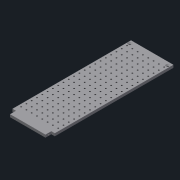
# Autodesk Inventor part: Mounting plate
Saved by Autodesk Inventor 2021.1 (Build 251245000, 245)
## iProperties
Created: 2020-05-07
Part Number: Mounting plate
Material: Generic
Document SubType Name: Modeling
Designer: Workshop Tech
Density: 1 g/cm^3
Appearance: Default
Author: Workshop Tech
Autodesk Inventor part; units mm, degrees
ref_plane "YZ Plane" through (0, 0, 0) normal (1, 0, 0) x (0, 1, 0)
ref_plane "XZ Plane" through (0, 0, 0) normal (0, 1, 0) x (-1, 0, 0)
ref_plane "XY Plane" through (0, 0, 0) normal (0, 0, 1) x (1, 0, 0)
sketch "Sketch1" plane through (0, 0, 0) normal (0, 1, 0) x (-1, 0, 0)
  line L0 (0, 0) -> (101.6, 0)
  line L1 (101.6, 0) -> (101.6, -298.45)
  line L2 (101.6, -298.45) -> (0, -298.45)
  line L3 (0, -298.45) -> (0, 0)
  dimension "d0" = 101.6
  dimension "d1" = 298.45
  constraints: 8 end point, 2 parallel, 1 horizontal, 1 perpendicular
  measures "d0" distance between parallel lines of L3 L1
  measures "d1" distance between parallel lines of L2 L0
extrude "Base" add sketch "Sketch1" along normal blind 6.35
sketch "Sketch7" plane through (0, 6.35, 0) normal (0, 1, 0) x (1, 0, 0)
  line L0 (0, 0) -> (0, 298.45) projected
  line L1 (-101.6, 0) -> (0, 0) projected
  line L2 (-101.6, 0) -> (0, 0) projected
  line L3 (0, 0) -> (0, 298.45) projected
  line L4 (0, 298.45) -> (-101.6, 298.45) projected
  line L5 (-101.6, 298.45) -> (-101.6, 0) projected
  point P0 (-95.25, 282.575)
  dimension "d35" = 15.875
  dimension "d36" = 6.35
  measures "d35" distance from line of L4 point (-95.25, 282.575)
  measures "d36" distance from line of L5 point (-95.25, 282.575)
hole "Threaded Mount Holes" at (-95.25, 6.35, -282.575) direction (0, -1, 0) diameter 3.242 end through all thread size "M4x0.7" class "6H" standard "ANSI Metric M Profile"
pattern_linear "Threaded Holes" count 21 spacing 12.7 along (0, 0, 1) count 8 spacing 12.7 along (1, 0, 0) of "Threaded Mount Holes"
sketch "Sketch8" plane through (0, 6.35, 0) normal (0, 1, 0) x (1, 0, 0)
  line L0 (0, 298.45) -> (-101.6, 298.45) projected
  line L1 (-101.6, 298.45) -> (-101.6, 0) projected
  point P0 (0, 0)
  point P1 (-96.4184, 290.703)
  dimension "d50" = 7.747
  dimension "d51" = 5.1816
  measures "d50" distance from line of L0 point (-96.418, 290.703)
  measures "d51" distance from line of point (-96.418, 290.703) L1
hole "Leg Mount Holes" at (-96.4184, 6.35, -290.703) direction (0, -1, 0) diameter 4.2926 end through all countersink diameter 9.398 countersink angle 90 clearance for "Countersunk Flat Head Screw ISO 2009/7046" size "M4" standard "ISO"
pattern_linear "Rectangular Pattern2" count 2 spacing 91.2368 along (1, 0, 0) of "Leg Mount Holes"
sketch "Sketch9" plane through (0, 6.35, 0) normal (0, 1, 0) x (1, 0, 0)
  line L0 (-101.6, 0) -> (0, 0) projected
  line L1 (-101.6, 0) -> (-93.2434, 0)
  line L2 (-93.2434, 0) -> (-93.2434, 14.097)
  line L3 (-93.2434, 14.097) -> (-101.6, 14.097)
  line L4 (-101.6, 14.097) -> (-101.6, 0)
  line L5 (0, 0) -> (-8.3566, 0)
  line L6 (-8.3566, 0) -> (-8.3566, 14.097)
  line L7 (-8.3566, 14.097) -> (0, 14.097)
  line L8 (0, 14.097) -> (0, 0)
  circle A0 centre (-96.4184, 290.703) radius 2.1463 projected
  line L9 (0, 298.45) -> (-101.6, 298.45) projected
  circle A1 centre (-5.1816, 290.703) radius 2.1463 projected
  dimension "d65" = 84.8868
  dimension "d66" = 8.3566
  dimension "d67" = 276.606
  dimension "d71" = 276.606
  constraints: 16 end point, 4 parallel, 2 horizontal, 2 perpendicular
  measures "d65" distance between parallel lines of L6 L2
  measures "d66" distance between parallel lines of L4 L2
  measures "d67" distance from line of A0.centre L3
  measures "d71" distance from line of L7 A1.centre
extrude "Leg Cut Out" cut sketch "Sketch9" against normal up to next contours L4 L3 L2 L0 | L6 L7 L8 L0
sketch "Sketch10" plane through (-8.3566, 6.35, 0) normal (1, 0, 0) x (0, 0, -1)
  line L0 (14.097, 0) -> (14.097, -6.35) projected
  line L1 (14.097, -6.35) -> (0, -6.35) projected
  point P0 (7.747, -3.175)
  dimension "d74" = 6.35
  dimension "d75" = 3.175
  measures "d74" distance from line of point (7.747, -3.175) L0
  measures "d75" distance from line of L1 point (7.747, -3.175)
hole "Leg Mount Hole 1" at (-8.3566, 3.175, -7.747) direction (-1, 0, 0) diameter 3.2512 depth 25.4 tip angle 118 countersink diameter 4.572 countersink angle 90
sketch "Sketch11" plane through (-93.2434, 6.35, -14.097) normal (-1, 0, 0) x (0, 0, 1)
  line L0 (0, -6.35) -> (0, 0) projected
  line L1 (14.097, -6.35) -> (0, -6.35) projected
  point P0 (6.35, -3.175)
  dimension "d83" = 6.35
  dimension "d84" = 3.175
  measures "d83" distance from line of L0 point (6.35, -3.175)
  measures "d84" distance from line of L1 point (6.35, -3.175)
hole "Leg Mount Hole 2" at (-93.2434, 3.175, -7.747) direction (1, 0, 0) diameter 3.2512 depth 25.4 tip angle 118 countersink diameter 4.572 countersink angle 90
body "Solid1"
